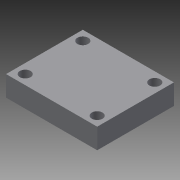
# Autodesk Inventor part: スペーサ改
Saved by Autodesk Inventor 2015 (Build 190159000, 159)
## iProperties
Created: 2013-10-24
Part Number: スペーサ改
Material: 一般
Document SubType Name: Modeling
Designer: kenta
Density: 1 g/cm^3
Appearance: 既定
Author: kenta
Autodesk Inventor part; units mm, degrees
ref_plane "YZ Plane" through (0, 0, 0) normal (1, 0, 0) x (0, 1, 0)
ref_plane "XZ Plane" through (0, 0, 0) normal (0, 1, 0) x (-1, 0, 0)
ref_plane "XY Plane" through (0, 0, 0) normal (0, 0, 1) x (1, 0, 0)
sketch "スケッチ1" plane through (0, 0, 0) normal (0, 0, 1) x (1, 0, 0)
  line L0 (-19, 16) -> (19, 16)
  line L1 (19, 16) -> (19, -16)
  line L2 (19, -16) -> (-19, -16)
  line L3 (-19, -16) -> (-19, 16)
  line L4 (-19, 16) -> (19, -16) construction
  line L5 (19, 16) -> (-19, -16) construction
  point P0 (0, 0)
  dimension "d0" = 38
  dimension "d2" = 32
  constraints: 12 end point, 2 midpoint, 2 parallel, 1 horizontal, 1 perpendicular
  measures "d0" distance between parallel lines of L1 L3
  measures "d2" distance between parallel lines of L2 L0
extrude "押し出し1" add sketch "スケッチ1" along normal blind 8.5
sketch "スケッチ2" plane through (0, 0, 8.5) normal (0, 0, 1) x (1, 0, 0)
  line L0 (19, 16) -> (-19, 16) projected
  line L1 (-19, 16) -> (-19, -16) projected
  line L2 (-19, -16) -> (19, -16) projected
  line L3 (19, -16) -> (19, 16) projected
  point P0 (0, 0)
  point P1 (-15, 12)
  point P2 (-15, -12)
  point P3 (15, -12)
  point P4 (15, 12)
  dimension "d5" = 4
  dimension "d6" = 4
  dimension "d7" = 4
  dimension "d8" = 4
  dimension "d9" = 4
  dimension "d10" = 4
  constraints: 2 horizontal alignment
  measures "d5" distance from line of L1 point (-15, 12)
  measures "d6" distance from line of L0 point (-15, 12)
  measures "d7" distance from line of L1 point (-15, -12)
  measures "d8" distance from line of point (-15, -12) L2
  measures "d9" distance from line of L3 point (15, 12)
  measures "d10" distance from line of L3 point (15, -12)
hole "穴1" at (-15, 12, 8.5) at (-15, -12, 8.5) at (15, -12, 8.5) at (15, 12, 8.5) direction (0, 0, -1) diameter 4.5 end through all
